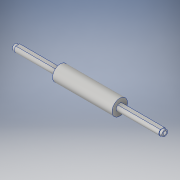
# Autodesk Inventor part: Belt Axle
Saved by Autodesk Inventor 2019.4 (Build 234330000, 330)
## iProperties
Created: 2020-01-11
Part Number: Belt Axle
Material: Aluminum 6061
Document SubType Name: Modeling
Designer: admin
Density: 2.7 g/cm^3
Appearance: Aluminum - Flat
Mass: 50.0907 g
Surface Area: 137.201 cm^2
Volume: 18.5521 cm^3
Author: admin
Autodesk Inventor part; units mm, degrees
ref_plane "YZ Plane" through (0, 0, 0) normal (1, 0, 0) x (0, 1, 0)
ref_plane "XZ Plane" through (0, 0, 0) normal (0, 1, 0) x (-1, 0, 0)
ref_plane "XY Plane" through (0, 0, 0) normal (0, 0, 1) x (1, 0, 0)
sketch "Sketch1" plane through (0, 0, 0) normal (0, 0, 1) x (1, 0, 0)
  line L0 (0, 0) -> (0, 4.9)
  line L1 (0, 4.9) -> (4, 4.9)
  line L2 (4, 4.9) -> (4, 5.9)
  line L3 (247.2, 5.9) -> (247.2, 4.9)
  line L4 (247.2, 4.9) -> (251.2, 4.9)
  line L5 (251.2, 4.9) -> (251.2, 0)
  line L6 (251.2, 0) -> (0, 0)
  line L7 (4, 5.9) -> (75.6, 5.9)
  line L8 (75.6, 5.9) -> (75.6, 13)
  line L9 (75.6, 13) -> (175.6, 13)
  line L10 (175.6, 13) -> (175.6, 5.9)
  line L11 (175.6, 5.9) -> (247.2, 5.9)
  dimension "d0" = 4.9
  dimension "d2" = 4
  dimension "d3" = 243.2
  dimension "d4" = 4
  dimension "d15" = 13
  dimension "d16" = 100
  dimension "d17" = 5.9
  constraints: 24 end point, 7 perpendicular, 3 point on line, 1 collinear, 1 horizontal, 1 parallel, 1 vertical
  measures "d0" distance between parallel lines of L6 L1
  measures "d2" distance of L3.end L4.end
  measures "d3" distance of L2.end L3.start
  measures "d4" distance of L0.end L1.end
  measures "d15" distance between parallel lines of L6 L9
  measures "d16" distance of L8.end L9.end
  measures "d17" distance between parallel lines of L6 L7
revolve "Revolution1" add sketch "Sketch1" angle 360 about axis through (251.2, 0, 0) along (-1, 0, 0)
sketch "Sketch2" plane through (247.2, 0, 0) normal (1, 0, 0) x (0, 0, -1)
  circle A0 centre (0, 0) radius 5.9 projected
  line L0 (-3.2863, 4.9) -> (3.2863, 4.9)
  circle A1 centre (0, 0) radius 4.9 projected
  constraints: 2 end point, 2 point on circle, 1 horizontal, 1 tangent
extrude "Extrusion1" cut sketch "Sketch2" against normal through all contours L0 A0 picked at (1.778, 5.1111)
sketch "Sketch3" plane through (251.2, 0, 0) normal (1, 0, 0) x (0, 0, -1)
  circle A0 centre (0, 0) radius 4.9 projected
  constraints: 1 coincident
hole "Hole1" at (251.2, 0, 0) direction (-1, 0, 0) diameter 6 end through all
body "Solid1"
